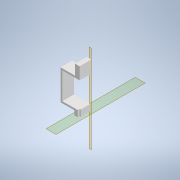
# Autodesk Inventor part: Battery
Saved by Autodesk Inventor 2020 (Build 240168000, 168)
## iProperties
Created: 2022-10-25
Part Number: Battery
Material: 일반
Document SubType Name: Modeling
Designer: ASUS
Density: 1 g/cm^3
Appearance: 기본값
Author: ASUS
Autodesk Inventor part; units mm, degrees
ref_plane "YZ Plane" through (0, 0, 0) normal (1, 0, 0) x (0, 1, 0)
ref_plane "XZ Plane" through (0, 0, 0) normal (0, 1, 0) x (-1, 0, 0)
ref_plane "XY Plane" through (0, 0, 0) normal (0, 0, 1) x (1, 0, 0)
ref_plane "작업 평면1" through (0, 0, 0) normal (0, 0, 1) x (1, 0, 0)
sketch "스케치1" plane through (0, 0, 0) normal (0, 0, 1) x (1, 0, 0)
  line L0 (-25.3, 192.5) -> (-25.3, 242.5)
  line L1 (-25.3, 192.5) -> (-25.3, 162)
  line L2 (0, -188.5) -> (0, 261.5) projected
  line L3 (0, -188.5) -> (0, 261.5) projected
  line L4 (-25.3, 228.54) -> (-13, 228.54)
  line L5 (0, -188.5) -> (0, 261.5) projected
  line L6 (-30, 10) -> (-97, 10)
  line L7 (-30, 10) -> (0, 10)
  line L8 (-30, -25) -> (-5, -25)
  line L9 (-30, -188.5) -> (-30, 261.5)
  line L10 (0, -188.5) -> (0, 261.5) projected
  line L11 (0, -188.5) -> (0, 261.5) projected
  line L12 (0, -188.5) -> (0, 261.5) projected
  line L13 (0, -188.5) -> (0, 261.5) projected
  line L14 (0, -188.5) -> (0, 261.5) projected
  line L15 (-13, 228.54) -> (0, 228.54) projected
  line L16 (0, -188.5) -> (0, 261.5) projected
  line L17 (-30, -188.5) -> (-30, 261.5)
  line L18 (-97, 0) -> (-97, 152)
  line L19 (-107, 152) -> (-107, 0)
  line L20 (-107, 0) -> (-97, 0)
  line L21 (-97, 0) -> (-30, 0)
  line L22 (-30, 10) -> (-97, 10)
  line L23 (-30, -188.5) -> (-30, 261.5)
  line L24 (-30, 10) -> (0, 10)
  line L25 (-18, -188.5) -> (-18, 261.5) projected
  line L26 (-22, 0) -> (-22, -188.5) projected
  line L27 (-5, -25) -> (0, -25) projected
  line L28 (-107, 152) -> (-107, 162)
  line L29 (-5, 0) -> (-5, -25) projected
  line L30 (0, 170.2) -> (-107, 170.2)
  line L31 (-107, 170.2) -> (-107, 160.2)
  line L32 (-107, 160.2) -> (0, 160.2)
  line L33 (0, 160.2) -> (0, 170.2)
  line L34 (-97, 152) -> (-97, 160.2)
  point P0 (0, 0)
  point P1 (0, 152)
  point P2 (0, 162)
  point P3 (0, 160.2)
  point P4 (-25.3, 170.2)
  dimension "d16" = 10
  dimension "d17" = 150.2
  constraints: 42 end point, 9 horizontal, 8 vertical, 3 point on line, 2 parallel, 2 perpendicular, 21 other
  measures "d16" distance of L31.end L30.end
  measures "d17" distance between parallel lines of L6 L32
extrude "돌출1" add sketch "스케치1" along normal blind 67 contours L0 L4 L25 L30 L1 | L30 L25 L32 L9 | L4 L15 L2 L30 L25 | L30 L2 L32 L25 | L9 L32 L28 L31 L30 | L25 L8 L9 L7 | L7 L2 L27 L8 L25 | L9 L21 L18 L6 | L34 L18 L20 L19 L28 L32
ref_plane "작업 평면2" through (-15.5, -25, -154) normal (0, -1, 0) x (1, 0, 0)
sketch "스케치2" plane through (-15.5, -25, -154) normal (0, -1, 0) x (1, 0, 0)
  line L0 (15.5, 104) -> (15.5, 74) projected
  line L1 (15.5, 74) -> (10.5, 74) projected
  line L2 (10.5, 74) -> (10.5, 18.5) projected
  line L3 (10.5, 18.5) -> (15.5, 18.5) projected
  line L4 (15.5, 18.5) -> (15.5, -6.5) projected
  line L5 (15.5, -6.5) -> (10.5, -6.5) projected
  line L6 (10.5, -6.5) -> (-9.5, -26.5) projected
  line L7 (-9.5, -26.5) -> (-19.5, -26.5) projected
  line L8 (-19.5, -26.5) -> (-19.5, -41.5) projected
  line L9 (-19.5, -41.5) -> (-25.5, -41.5) projected
  line L10 (-25.5, -41.5) -> (-25.5, -46.5) projected
  line L11 (-25.5, -46.5) -> (-22.5, -46.5) projected
  line L12 (-22.5, -46.5) -> (-22.5, -71.5) projected
  line L13 (-22.5, -71.5) -> (-25.5, -71.5) projected
  line L14 (-25.5, -71.5) -> (-25.5, -78) projected
  line L15 (-25.5, -78) -> (-22.5, -78) projected
  line L16 (-22.5, -78) -> (-22.5, -114) projected
  line L17 (-22.5, -114) -> (-7.5, -114) projected
  line L18 (-7.5, -114) -> (-7.5, -44) projected
  line L19 (-7.5, -44) -> (25.5, -11) projected
  line L20 (25.5, -11) -> (25.5, 239) projected
  line L21 (25.5, 239) -> (-7.5, 272) projected
  line L22 (-7.5, 272) -> (-7.5, 342) projected
  line L23 (-7.5, 342) -> (-22.5, 342) projected
  line L24 (-22.5, 342) -> (-22.5, 306) projected
  line L25 (-22.5, 306) -> (-25.5, 306) projected
  line L26 (-25.5, 306) -> (-25.5, 299.5) projected
  line L27 (-25.5, 299.5) -> (-22.5, 299.5) projected
  line L28 (-22.5, 299.5) -> (-22.5, 274.5) projected
  line L29 (-22.5, 274.5) -> (-25.5, 274.5) projected
  line L30 (-25.5, 274.5) -> (-25.5, 269.5) projected
  line L31 (-25.5, 269.5) -> (-19.5, 269.5) projected
  line L32 (-19.5, 269.5) -> (-19.5, 254.5) projected
  line L33 (-19.5, 254.5) -> (-9.5, 254.5) projected
  line L34 (-9.5, 254.5) -> (10.5, 234.5) projected
  line L35 (10.5, 234.5) -> (15.5, 234.5) projected
  line L36 (15.5, 234.5) -> (15.5, 209.5) projected
  line L37 (15.5, 209.5) -> (10.5, 209.5) projected
  line L38 (10.5, 209.5) -> (10.5, 154) projected
  line L39 (10.5, 154) -> (15.5, 154) projected
  line L40 (15.5, 154) -> (15.5, 124) projected
  line L41 (15.5, 124) -> (10.5, 124) projected
  line L42 (10.5, 124) -> (10.5, 104) projected
  line L43 (10.5, 104) -> (15.5, 104) projected
  line L44 (15.5, 124) -> (15.5, 104)
  line L45 (15.5, 154) -> (15.5, 221) projected
  line L46 (-14.5, 154) -> (15.5, 154) projected
  line L47 (15.5, 154) -> (15.5, 221) projected
  line L48 (-14.5, 221) -> (15.5, 221) projected
  line L49 (-14.5, 154) -> (-14.5, 221) projected
  line L50 (5.5, 209.5) -> (15.5, 209.5) projected
  line L51 (5.5, 209.5) -> (5.5, 221)
  line L52 (-14.5, 221) -> (15.5, 221) projected
  point P0 (15.5, 221)
  constraints: 4 end point, 2 perpendicular, 1 point on line
extrude "돌출2" cut sketch "스케치2" against normal blind 67 contours L39 L38 L37 L45 | L37 L50 L51 L48 L36
sketch "스케치6" plane through (-25.3, 162, 0) normal (-1, 0, 0) x (0, 0, 1)
  line L0 (230, 48.5399) -> (-310, 48.5399) projected
  line L1 (230, 54.5399) -> (-310, 54.5399) projected
  line L2 (0, 8.2) -> (0, -162) projected
  line L3 (0, -162) -> (67, -162) projected
  line L4 (67, 8.2) -> (67, -162) projected
  line L5 (0, 66.54) -> (0, 8.2) projected
  line L6 (67, 66.54) -> (67, 8.2) projected
  line L7 (0, 66.54) -> (67, 66.54) projected
  line L8 (67, 66.54) -> (67, 0) projected
  line L9 (67, 54.5399) -> (67, 48.5399)
  line L10 (0, 8.2) -> (67, 8.2) projected
  line L11 (0, 8.2) -> (67, 8.2) projected
  point P0 (0, -162)
  point P1 (67, 0)
  point P2 (54, 51.5399)
  point P3 (13, 51.5399)
  point P4 (67, 51.5399)
  dimension "d7" = 13
  dimension "d8" = 13
  constraints: 4 point on line, 2 end point, 2 horizontal alignment, 1 midpoint
  measures "d7" distance of point (67, 51.54) point (54, 51.54)
  measures "d8" distance from line of L5 point (13, 51.54)
hole "구멍1" at (-25.3, 213.5399, 54) at (-25.3, 213.5399, 13) direction (1, 0, 0) diameter 4.5 end through all counterbore diameter 8 counterbore depth 4.6 clearance for "Socket Head Cap Screw ISO 4762" size "M4" standard "ISO"
sketch "스케치9" plane through (0, 160.2, 0) normal (1, 0, 0) x (0, 0, -1)
  circle A0 centre (-33.5, 21.15) radius 2.25 projected
  point P0 (0, -160.2)
hole "구멍2" at (0, 181.35, 33.5) direction (-1, 0, 0) diameter 4.5 end through all counterbore diameter 8 counterbore depth 8 clearance for "Socket Head Cap Screw ISO 4762" size "M4" standard "ISO"
sketch "스케치10" plane through (0, 0, 67) normal (0, 0, 1) x (1, 0, 0)
  line L0 (-10, -25) -> (-10, 10) projected
  line L1 (-10, 10) -> (-97, 10) projected
  line L2 (-97, 10) -> (-97, 160.2) projected
  line L3 (-97, 160.2) -> (0, 160.2) projected
  line L4 (0, 160.2) -> (0, 228.54) projected
  line L5 (0, 228.54) -> (-25.3, 228.54) projected
  line L6 (-25.3, 228.54) -> (-25.3, 170.2) projected
  line L7 (-25.3, 170.2) -> (-107, 170.2) projected
  line L8 (-107, 170.2) -> (-107, 0) projected
  line L9 (-107, 0) -> (-30, 0) projected
  line L10 (-30, 0) -> (-30, -25) projected
  line L11 (-30, -25) -> (-10, -25) projected
  point P0 (0, 0)
extrude "돌출4" cut sketch "스케치10" against normal blind 1
